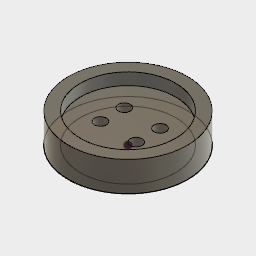
fastener (Autodesk Fusion 360 design; units mm, degrees)
Autodesk Fusion 360 part; units mm, degrees
sketch "草图1" plane through (0, 0, 0) normal (0, 1, 0) x (1, 0, 0)
  circle A0 centre (0, 0) radius 10
  circle A1 centre (0, 0) radius 8
  dimension "d1" = 20
  dimension "d2" = 2
  measures "d1" diameter of A0
extrude "拉伸1" add sketch "草图1" along normal blind 3 contours A1 makes body 1
extrude "拉伸2" add sketch "草图1" along normal blind 5 bodies 1
cylinder "圆柱体基本要素1" add diameter 2 height 20 placed x (1, 0, 0) y (0, 0, -1) z (0, 1, 0) at (15, 0, 30) separate body makes body 2
move_body "移动1" bodies 2 to x (1, 0, 0) y (0, 1, 0) z (0, 0, 1) at (-15.0005, 0.0913, -29.9153)
move_body "移动2" bodies 2 to x (1, 0, 0) y (0, 1, 0) z (0, 0, 1) at (0, 0, -0.0913)
move_body "移动3" bodies 2 to x (1, 0, 0) y (0, 1, 0) z (0, 0, 1) at (24.0594, 0, -2.9322)
move_body "移动4" bodies 2 to x (1, 0, 0) y (0, 1, 0) z (0, 0, 1) at (-20.7863, 0, 5.8274)
pattern_linear "R-阵列1" count 2 spacing 6 along (1, 0, 0) count 2 spacing 4 along (0, 0, 1) of bodies 2 makes body 3 at (10.2676, 13.4246, 2.9882) makes body 4 at (4.2676, 13.4246, 6.9882) makes body 5 at (10.2676, 13.4246, 6.9882)
move_body "移动5" bodies 2 3 5 4 to x (1, 0, 0) y (0, 1, 0) z (0, 0, 1) at (-5.932, -2.5575, -4.9286)
move_body "移动6" bodies 2 3 5 4 to x (1, 0, 0) y (0, 1, 0) z (0, 0, 1) at (-0.0913, 0, -0.0913)
combine "合并1" operation cut target body 1 tool bodies 2 3 4 5
